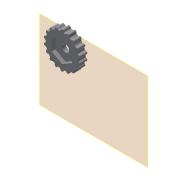
# Autodesk Inventor part: cellSTORM_v5_chiptray_adjustmentscrew
Saved by Autodesk Inventor 2019.4 (Build 234330000, 330)
## iProperties
Created: 2020-08-17
Part Number: cellSTORM_v5_chiptray_adjustmentscrew
Material: Generic
Document SubType Name: Modeling
Designer: diederichbenedict
Density: 1 g/cm^3
Appearance: Default
Author: diederichbenedict
Autodesk Inventor part; units mm, degrees
ref_plane "YZ Plane" through (0, 0, 0) normal (1, 0, 0) x (0, 1, 0)
ref_plane "XZ Plane" through (0, 0, 0) normal (0, 1, 0) x (-1, 0, 0)
ref_plane "XY Plane" through (0, 0, 0) normal (0, 0, 1) x (1, 0, 0)
ref_plane "Work Plane1" through (0, 0, 0) normal (0, 0, 1) x (1, 0, 0)
sketch "Sketch1" plane through (0, 0, 0) normal (0, 0, 1) x (1, 0, 0)
  circle A0 centre (-16.5191, 0.5183) radius 1.4 projected
  circle A1 centre (-9.7905, 10.5) radius 2.95 construction
  circle A2 centre (14.4582, 10.5) radius 2.95 projected
  circle A3 centre (2.3338, -10.5) radius 2.95 projected
  line L0 (19.7905, 14.5) -> (19.7905, -14.5) projected
  line L1 (-19.7905, 14.5) -> (19.7905, 14.5) projected
  line L2 (-19.7905, -14.5) -> (-19.7905, 14.5) projected
  line L3 (19.7905, -14.5) -> (-19.7905, -14.5) projected
  circle A4 centre (-9.7905, 10.5) radius 1.5 construction
  circle A5 centre (-9.7905, 10.5) radius 6.5
  circle A6 centre (-9.7905, 10.5) radius 1.4
  point P0 (0, 0)
  dimension "d0" = 13
  dimension "d1" = 2.8
  constraints: 2 centre point, 2 coincident
  measures "d0" diameter of A5
  measures "d1" diameter of A6
extrude "Extrusion1" add sketch "Sketch1" along normal blind 3 contours A5 L1 | L1 A5
sketch "Sketch2" plane through (-9.7905, 10.5, 3) normal (0, 0, 1) x (1, 0, 0)
  circle A0 centre (0, 0) radius 1.4 projected
  circle A1 centre (0, 0) radius 6.5 projected
  circle A2 centre (0, 0) radius 6.5 projected
  line L0 (0, 6.5) -> (0, 8)
  line L1 (0, 8) -> (0.718, 6.4602)
  arc A3 (0.718, 6.4602) -> (0, 6.5) centre (0, 0) ccw
  line L2 (0, 8) -> (-0.718, 6.4602)
  arc A4 (0, 6.5) -> (-0.718, 6.4602) centre (0, 0) ccw
  point P0 (9.7905, -10.5)
  dimension "d4" = 1.5
  dimension "d5" = 25
  constraints: 6 end point, 6 point on circle, 2 centre point, 1 concentric, 1 symmetric about line, 1 vertical, 1 other
  measures "d4" distance of L0.start L0.end
  measures "d5" angle of L0 L1
extrude "Extrusion2" add sketch "Sketch2" against normal up to surface (3 mm away) contours A1 L0 L1 | L2 L0 A1
fillet "Fillet1" radius 0.5 3 edges at (-9.7905, 18.5, 1.5) (-10.5085, 16.9602, 1.5) (-9.0725, 16.9602, 1.5)
pattern_circular "Circular Pattern1" count 18 over 360 about axis through (-9.7905, 10.5, 0) along (0, 0, 1) of "Extrusion2", "Fillet1"
sketch "Sketch3" plane through (0, 0, 3) normal (0, 0, 1) x (1, 0, 0)
  circle A0 centre (-9.7905, 10.5) radius 1.4 projected
  arc A1 (-6.9609, 16.9494) -> (-7.8125, 17.2593) centre (-7.459, 16.9058) ccw projected
  line L0 (-8.0618, 17.0101) -> (-7.8125, 17.2593) projected
  arc A2 (-8.5136, 16.8733) -> (-8.0618, 17.0101) centre (-8.4154, 17.3636) ccw projected
  arc A3 (-8.5136, 16.8733) -> (-8.8106, 16.9257) centre (-9.7905, 10.5) ccw projected
  arc A4 (-9.1884, 17.2087) -> (-8.8106, 16.9257) centre (-8.7352, 17.42) ccw projected
  line L1 (-9.3374, 17.5282) -> (-9.1884, 17.2087) projected
  arc A5 (-9.3374, 17.5282) -> (-10.2437, 17.5282) centre (-9.7905, 17.3169) ccw projected
  line L2 (-10.3927, 17.2087) -> (-10.2437, 17.5282) projected
  arc A6 (-10.7704, 16.9257) -> (-10.3927, 17.2087) centre (-10.8458, 17.42) ccw projected
  arc A7 (-10.7704, 16.9257) -> (-11.0674, 16.8733) centre (-9.7905, 10.5) ccw projected
  arc A8 (-11.5192, 17.0101) -> (-11.0674, 16.8733) centre (-11.1656, 17.3636) ccw projected
  line L3 (-11.7685, 17.2593) -> (-11.5192, 17.0101) projected
  arc A9 (-11.7685, 17.2593) -> (-12.6201, 16.9494) centre (-12.122, 16.9058) ccw projected
  line L4 (-12.6509, 16.5982) -> (-12.6201, 16.9494) projected
  arc A10 (-12.9091, 16.203) -> (-12.6509, 16.5982) centre (-13.1489, 16.6417) ccw projected
  arc A11 (-12.9091, 16.203) -> (-13.1702, 16.0523) centre (-9.7905, 10.5) ccw projected
  arc A12 (-13.6415, 16.0262) -> (-13.1702, 16.0523) centre (-13.4302, 16.4794) ccw projected
  line L5 (-13.961, 16.1752) -> (-13.6415, 16.0262) projected
  arc A13 (-13.961, 16.1752) -> (-14.6553, 15.5926) centre (-14.1723, 15.722) ccw projected
  line L6 (-14.564, 15.2521) -> (-14.6553, 15.5926) projected
  arc A14 (-14.6715, 14.7925) -> (-14.564, 15.2521) centre (-15.047, 15.1227) ccw projected
  arc A15 (-14.6715, 14.7925) -> (-14.8654, 14.5615) centre (-9.7905, 10.5) ccw projected
  arc A16 (-15.2993, 14.3758) -> (-14.8654, 14.5615) centre (-15.2557, 14.8739) ccw projected
  line L7 (-15.6505, 14.4065) -> (-15.2993, 14.3758) projected
  arc A17 (-15.6505, 14.4065) -> (-16.1037, 13.6217) centre (-15.6941, 13.9084) ccw projected
  line L8 (-15.9015, 13.3329) -> (-16.1037, 13.6217) projected
  arc A18 (-15.8453, 12.8642) -> (-15.9015, 13.3329) centre (-16.3111, 13.0461) ccw projected
  arc A19 (-15.8453, 12.8642) -> (-15.9484, 12.5809) centre (-9.7905, 10.5) ccw projected
  arc A20 (-16.2927, 12.258) -> (-15.9484, 12.5809) centre (-16.4221, 12.7409) ccw projected
  line L9 (-16.6333, 12.1667) -> (-16.2927, 12.258) projected
  arc A21 (-16.6333, 12.1667) -> (-16.7906, 11.2742) centre (-16.5038, 11.6837) ccw projected
  line L10 (-16.5018, 11.0719) -> (-16.7906, 11.2742) projected
  arc A22 (-16.2888, 10.6508) -> (-16.5018, 11.0719) centre (-16.7886, 10.6624) ccw projected
  arc A23 (-16.2888, 10.6508) -> (-16.2888, 10.3492) centre (-9.7905, 10.5) ccw projected
  arc A24 (-16.5018, 9.9281) -> (-16.2888, 10.3492) centre (-16.7886, 10.3376) ccw projected
  line L11 (-16.7906, 9.7258) -> (-16.5018, 9.9281) projected
  arc A25 (-16.7906, 9.7258) -> (-16.6333, 8.8333) centre (-16.5038, 9.3163) ccw projected
  line L12 (-16.2927, 8.742) -> (-16.6333, 8.8333) projected
  arc A26 (-15.9484, 8.4191) -> (-16.2927, 8.742) centre (-16.4221, 8.2591) ccw projected
  arc A27 (-15.9484, 8.4191) -> (-15.8453, 8.1358) centre (-9.7905, 10.5) ccw projected
  arc A28 (-15.9015, 7.6671) -> (-15.8453, 8.1358) centre (-16.3111, 7.9539) ccw projected
  line L13 (-16.1037, 7.3783) -> (-15.9015, 7.6671) projected
  arc A29 (-16.1037, 7.3783) -> (-15.6505, 6.5935) centre (-15.6941, 7.0916) ccw projected
  line L14 (-15.2993, 6.6242) -> (-15.6505, 6.5935) projected
  arc A30 (-14.8654, 6.4385) -> (-15.2993, 6.6242) centre (-15.2557, 6.1261) ccw projected
  arc A31 (-14.8654, 6.4385) -> (-14.6715, 6.2075) centre (-9.7905, 10.5) ccw projected
  arc A32 (-14.564, 5.7479) -> (-14.6715, 6.2075) centre (-15.047, 5.8773) ccw projected
  line L15 (-14.6553, 5.4074) -> (-14.564, 5.7479) projected
  arc A33 (-14.6553, 5.4074) -> (-13.961, 4.8248) centre (-14.1723, 5.278) ccw projected
  line L16 (-13.6415, 4.9738) -> (-13.961, 4.8248) projected
  arc A34 (-13.1702, 4.9477) -> (-13.6415, 4.9738) centre (-13.4302, 4.5206) ccw projected
  arc A35 (-13.1702, 4.9477) -> (-12.9091, 4.797) centre (-9.7905, 10.5) ccw projected
  arc A36 (-12.6509, 4.4018) -> (-12.9091, 4.797) centre (-13.1489, 4.3583) ccw projected
  line L17 (-12.6201, 4.0506) -> (-12.6509, 4.4018) projected
  arc A37 (-12.6201, 4.0506) -> (-11.7685, 3.7407) centre (-12.122, 4.0942) ccw projected
  line L18 (-11.5192, 3.9899) -> (-11.7685, 3.7407) projected
  arc A38 (-11.0674, 4.1267) -> (-11.5192, 3.9899) centre (-11.1656, 3.6364) ccw projected
  arc A39 (-11.0674, 4.1267) -> (-10.7704, 4.0743) centre (-9.7905, 10.5) ccw projected
  arc A40 (-10.3927, 3.7913) -> (-10.7704, 4.0743) centre (-10.8458, 3.58) ccw projected
  line L19 (-10.2437, 3.4718) -> (-10.3927, 3.7913) projected
  arc A41 (-10.2437, 3.4718) -> (-9.3374, 3.4718) centre (-9.7905, 3.6831) ccw projected
  line L20 (-9.1884, 3.7913) -> (-9.3374, 3.4718) projected
  arc A42 (-8.8106, 4.0743) -> (-9.1884, 3.7913) centre (-8.7352, 3.58) ccw projected
  arc A43 (-8.8106, 4.0743) -> (-8.5136, 4.1267) centre (-9.7905, 10.5) ccw projected
  arc A44 (-8.0618, 3.9899) -> (-8.5136, 4.1267) centre (-8.4154, 3.6364) ccw projected
  line L21 (-7.8125, 3.7407) -> (-8.0618, 3.9899) projected
  arc A45 (-7.8125, 3.7407) -> (-6.9609, 4.0506) centre (-7.459, 4.0942) ccw projected
  line L22 (-6.9302, 4.4018) -> (-6.9609, 4.0506) projected
  arc A46 (-6.672, 4.797) -> (-6.9302, 4.4018) centre (-6.4321, 4.3583) ccw projected
  arc A47 (-6.672, 4.797) -> (-6.4108, 4.9477) centre (-9.7905, 10.5) ccw projected
  arc A48 (-5.9395, 4.9738) -> (-6.4108, 4.9477) centre (-6.1508, 4.5206) ccw projected
  line L23 (-5.62, 4.8248) -> (-5.9395, 4.9738) projected
  arc A49 (-5.62, 4.8248) -> (-4.9257, 5.4074) centre (-5.4087, 5.278) ccw projected
  line L24 (-5.017, 5.7479) -> (-4.9257, 5.4074) projected
  arc A50 (-4.9095, 6.2075) -> (-5.017, 5.7479) centre (-4.534, 5.8773) ccw projected
  arc A51 (-4.9095, 6.2075) -> (-4.7156, 6.4385) centre (-9.7905, 10.5) ccw projected
  arc A52 (-4.2817, 6.6242) -> (-4.7156, 6.4385) centre (-4.3253, 6.1261) ccw projected
  line L25 (-3.9305, 6.5935) -> (-4.2817, 6.6242) projected
  arc A53 (-3.9305, 6.5935) -> (-3.4773, 7.3783) centre (-3.8869, 7.0916) ccw projected
  line L26 (-3.6795, 7.6671) -> (-3.4773, 7.3783) projected
  arc A54 (-3.7357, 8.1358) -> (-3.6795, 7.6671) centre (-3.27, 7.9539) ccw projected
  arc A55 (-3.7357, 8.1358) -> (-3.6326, 8.4191) centre (-9.7905, 10.5) ccw projected
  arc A56 (-3.2883, 8.742) -> (-3.6326, 8.4191) centre (-3.1589, 8.2591) ccw projected
  line L27 (-2.9478, 8.8333) -> (-3.2883, 8.742) projected
  arc A57 (-2.9478, 8.8333) -> (-2.7904, 9.7258) centre (-3.0772, 9.3163) ccw projected
  line L28 (-3.0792, 9.9281) -> (-2.7904, 9.7258) projected
  arc A58 (-3.2923, 10.3492) -> (-3.0792, 9.9281) centre (-2.7924, 10.3376) ccw projected
  arc A59 (-3.2923, 10.3492) -> (-3.2923, 10.6508) centre (-9.7905, 10.5) ccw projected
  arc A60 (-3.0792, 11.0719) -> (-3.2923, 10.6508) centre (-2.7924, 10.6624) ccw projected
  line L29 (-2.7904, 11.2742) -> (-3.0792, 11.0719) projected
  arc A61 (-2.7904, 11.2742) -> (-2.9478, 12.1667) centre (-3.0772, 11.6837) ccw projected
  line L30 (-3.2883, 12.258) -> (-2.9478, 12.1667) projected
  arc A62 (-3.6326, 12.5809) -> (-3.2883, 12.258) centre (-3.1589, 12.7409) ccw projected
  arc A63 (-3.6326, 12.5809) -> (-3.7357, 12.8642) centre (-9.7905, 10.5) ccw projected
  arc A64 (-3.6795, 13.3329) -> (-3.7357, 12.8642) centre (-3.27, 13.0461) ccw projected
  line L31 (-3.4773, 13.6217) -> (-3.6795, 13.3329) projected
  arc A65 (-3.4773, 13.6217) -> (-3.9305, 14.4065) centre (-3.8869, 13.9084) ccw projected
  line L32 (-4.2817, 14.3758) -> (-3.9305, 14.4065) projected
  arc A66 (-4.7156, 14.5615) -> (-4.2817, 14.3758) centre (-4.3253, 14.8739) ccw projected
  arc A67 (-4.7156, 14.5615) -> (-4.9095, 14.7925) centre (-9.7905, 10.5) ccw projected
  arc A68 (-5.017, 15.2521) -> (-4.9095, 14.7925) centre (-4.534, 15.1227) ccw projected
  line L33 (-4.9257, 15.5926) -> (-5.017, 15.2521) projected
  arc A69 (-4.9257, 15.5926) -> (-5.62, 16.1752) centre (-5.4087, 15.722) ccw projected
  line L34 (-5.9395, 16.0262) -> (-5.62, 16.1752) projected
  arc A70 (-6.4108, 16.0523) -> (-5.9395, 16.0262) centre (-6.1508, 16.4794) ccw projected
  arc A71 (-6.4108, 16.0523) -> (-6.672, 16.203) centre (-9.7905, 10.5) ccw projected
  arc A72 (-6.9302, 16.5982) -> (-6.672, 16.203) centre (-6.4321, 16.6417) ccw projected
  line L35 (-6.9609, 16.9494) -> (-6.9302, 16.5982) projected
  line L36 (-13.8405, 8.1617) -> (-13.8405, 12.8383)
  line L37 (-13.8405, 12.8383) -> (-9.7905, 15.1765)
  line L38 (-9.7905, 15.1765) -> (-5.7405, 12.8383)
  line L39 (-5.7405, 12.8383) -> (-5.7405, 8.1617)
  line L40 (-5.7405, 8.1617) -> (-9.7905, 5.8235)
  line L41 (-9.7905, 5.8235) -> (-13.8405, 8.1617)
  line L42 (0, 21.3803) -> (0, -3.5634) projected
  point P0 (0, 0)
  dimension "d12" = 8.1
  constraints: 12 end point, 1 coincident, 1 parallel, 13 other
  measures "d12" distance between parallel lines of L36 L39
extrude "Extrusion3" cut sketch "Sketch3" against normal blind 1.5 contours L36 L37 L38 L39 L40 L41
body "Solid1"
